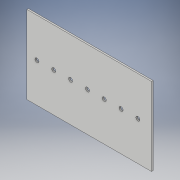
# Autodesk Inventor part: topgearbase
Saved by Autodesk Inventor 2018 (Build 220112000, 112)
## iProperties
Created: 2019-03-28
Part Number: topgearbase
Material: Generic
Document SubType Name: Modeling
Designer: F8PLTW
Density: 1 g/cm^3
Appearance: Default
Author: F8PLTW
Autodesk Inventor part; units mm, degrees
ref_plane "YZ Plane" through (0, 0, 0) normal (1, 0, 0) x (0, 1, 0)
ref_plane "XZ Plane" through (0, 0, 0) normal (0, 1, 0) x (-1, 0, 0)
ref_plane "XY Plane" through (0, 0, 0) normal (0, 0, 1) x (1, 0, 0)
sketch "Sketch1" plane through (0, 0, 0) normal (0, 0, 1) x (1, 0, 0)
  line L0 (-23.2495, 10.1907) -> (98.6705, 10.1907)
  line L1 (98.6705, 10.1907) -> (98.6705, -66.0093)
  line L2 (98.6705, -66.0093) -> (-23.2495, -66.0093)
  line L3 (-23.2495, -66.0093) -> (-23.2495, 10.1907)
  point P0 (0, 0)
  dimension "d0" = 121.92
  dimension "d1" = 76.2
  constraints: 8 end point, 2 parallel, 1 horizontal, 1 perpendicular
  measures "d0" distance of L1.end L2.end
  measures "d1" distance of L0.end L1.end
extrude "Extrusion1" add sketch "Sketch1" along normal blind 1.5875
sketch "Sketch2" plane through (0, 0, 1.5875) normal (0, 0, 1) x (1, 0, 0)
  circle A0 centre (-13.3114, -27.9093) radius 2
  circle A1 centre (3.1346, -27.9093) radius 2
  circle A2 centre (19.5806, -27.9093) radius 2
  circle A3 centre (36.0266, -27.9093) radius 2
  circle A4 centre (68.9186, -27.9093) radius 2
  circle A5 centre (85.3646, -27.9093) radius 2
  line L0 (98.6705, -66.0093) -> (98.6705, 10.1907) projected
  line L1 (68.9186, -27.9093) -> (51.2881, -27.9093) construction
  circle A6 centre (52.4726, -27.9093) radius 2
  point P0 (0, 0)
  dimension "d4" = 4
  dimension "d5" = 4
  dimension "d6" = 4
  dimension "d7" = 4
  dimension "d9" = 4
  dimension "d10" = 4
  dimension "d11" = 12.446
  dimension "d12" = 12.446
  dimension "d13" = 12.446
  dimension "d18" = 4
  dimension "d20" = 12.446
  dimension "d21" = 12.446
  dimension "d22" = 12.446
  constraints: 7 centre point, 2 end point, 1 horizontal, 1 point on line
  measures "d4" diameter of A0
  measures "d5" diameter of A1
  measures "d6" diameter of A2
  measures "d7" diameter of A3
  measures "d9" diameter of A4
  measures "d10" diameter of A5
  measures "d18" diameter of A6
extrude "Extrusion2" cut sketch "Sketch2" against normal blind 1.5875
body "Solid1"
